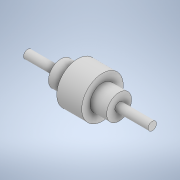
# Autodesk Inventor part: 零件1
Saved by Autodesk Inventor 2020 (Build 240168000, 168)
## iProperties
Created: 2020-12-28
Part Number: 零件1
Material: 一般
Document SubType Name: Modeling
Designer: User
Density: 1 g/cm^3
Appearance: 預設
Author: User
Autodesk Inventor part; units mm, degrees
ref_plane "YZ Plane" through (0, 0, 0) normal (1, 0, 0) x (0, 1, 0)
ref_plane "XZ Plane" through (0, 0, 0) normal (0, 1, 0) x (-1, 0, 0)
ref_plane "XY Plane" through (0, 0, 0) normal (0, 0, 1) x (1, 0, 0)
sketch "草圖1" plane through (0, 0, 0) normal (0, 0, 1) x (1, 0, 0)
  line L0 (0, 0) -> (0, 1270)
  line L1 (0, 1270) -> (1524, 1270)
  line L2 (1524, 1270) -> (1524, 0)
  line L3 (1524, 0) -> (1524, 762)
  line L4 (1524, 762) -> (2540, 762)
  line L5 (2540, 762) -> (2540, 0)
  line L6 (2540, 0) -> (2540, 254)
  line L7 (2540, 254) -> (4572, 254)
  line L8 (4572, 254) -> (4572, 0)
  line L9 (4572, 0) -> (0, 0)
  line L10 (762, 0) -> (762, 1270)
  line L11 (1524, 1270) -> (0, 1270)
  line L12 (0, 1270) -> (0, 0)
  line L13 (0, 0) -> (0, 762)
  line L14 (0, 762) -> (-1016, 762)
  line L15 (-1016, 762) -> (-1016, 0)
  line L16 (-1016, 0) -> (-1016, 254)
  line L17 (-1016, 254) -> (-3048, 254)
  line L18 (-3048, 254) -> (-3048, 0)
  line L19 (-3048, 0) -> (1524, 0)
  dimension "d0" = 1270
  dimension "d1" = 1524
  dimension "d2" = 762
  dimension "d3" = 1016
  dimension "d4" = 254
  dimension "d5" = 2032
  constraints: 40 end point, 10 symmetric about line, 7 perpendicular, 5 point on line, 1 midpoint, 1 vertical
  measures "d0" distance of L0.start L0.end
  measures "d1" distance of L0.end L1.end
  measures "d2" distance of L2.end L3.end
  measures "d3" distance of L3.end L4.end
  measures "d4" distance of L5.end L6.end
  measures "d5" distance of L6.end L7.end
revolve "迴轉1" add sketch "草圖1" angle 360 about axis through (-3048, 0, 0) along (1, 0, 0)
